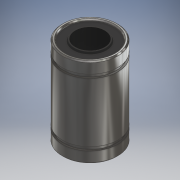
# Autodesk Inventor part: линейный подшипник 8х15х24
Saved by Autodesk Inventor 2017 (Build 210142000, 142)
## iProperties
Part Number: линейный подшипник 8х15х24
Material: Типовые
Document SubType Name: Modeling
Designer: Dota
Density: 1 g/cm^3
Appearance: Сталь — полированная
Author: Dota
Autodesk Inventor part; units mm, degrees
ref_plane "YZ Plane" through (0, 0, 0) normal (1, 0, 0) x (0, 1, 0)
ref_plane "XZ Plane" through (0, 0, 0) normal (0, 1, 0) x (-1, 0, 0)
ref_plane "XY Plane" through (0, 0, 0) normal (0, 0, 1) x (1, 0, 0)
sketch "Эскиз1" plane through (0, 0, 0) normal (0, 0, 1) x (1, 0, 0)
  circle A0 centre (0, 0) radius 4
  circle A1 centre (0, 0) radius 7.5
  circle A2 centre (0, 0) radius 6.5
  circle A3 centre (0, 0) radius 4.5
  circle A4 centre (0, 0) radius 7
  dimension "d0" = 8
  dimension "d1" = 15
  dimension "d2" = 1
  dimension "d3" = 0.5
  dimension "d25" = 0.5
  constraints: 5 centre point, 5 coincident
  measures "d0" diameter of A0
  measures "d1" diameter of A1
  measures "d2" radial gap between concentric circles of A2 A1
  measures "d3" radial gap between concentric circles of A0 A3
  measures "d25" radial gap between concentric circles of A1 A4
extrude "Выдавливание1" add sketch "Эскиз1" along normal mid plane 24 contours A3
extrude "Выдавливание2" add sketch "Эскиз1" along normal mid plane 23 contours A2
extrude "Выдавливание3" add sketch "Эскиз1" along normal mid plane 24 contours A1 | A4
chamfer "Фаска1" distance 0.3 angle 45 1 edges at (-6.5, 0, 12)
chamfer "Фаска2" distance 0.3 angle 45 1 edges at (-7.5, 0, 12)
chamfer "Фаска3" distance 0.3 angle 45 2 edges at (-7.5, 0, -12) (-6.5, 0, -12)
chamfer "Фаска4" distance 0.3 distance2 0.5 1 edges at (-4.5, 0, -12) measured on face at (4.251, -0.6781, -12)
chamfer "Фаска5" distance 0.3 distance2 0.5 1 edges at (-4.5, 0, 12) measured on face at (4.251, -0.6781, 12)
extrude "Выдавливание4" cut sketch "Эскиз1" along normal mid plane 18 contours A1
extrude "Выдавливание5" add sketch "Эскиз1" along normal mid plane 16 contours A1
